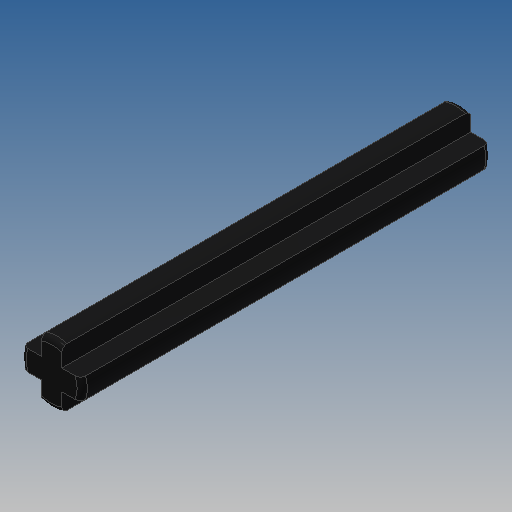
# Autodesk Inventor part: 3705-Black
Saved by Autodesk Inventor 2022.2 (Build 262287000, 287)
## iProperties
Created: 2014-06-05
Part Number: 3705-Black
Material: ABS Plastic
Document SubType Name: Modeling
Designer: D. Kohfeld
Density: 1.06 g/cm^3
Appearance: Black
Mass: 0.423877 g
Surface Area: 6.05529 cm^2
Volume: 0.399884 cm^3
Description: Technic, Axle 4
Author: D. Kohfeld
Autodesk Inventor part; units mm, degrees
ref_plane "YZ Plane" through (0, 0, 0) normal (1, 0, 0) x (0, 1, 0)
ref_plane "XZ Plane" through (0, 0, 0) normal (0, 1, 0) x (-1, 0, 0)
ref_plane "XY Plane" through (0, 0, 0) normal (0, 0, 1) x (1, 0, 0)
sketch "Sketch1" plane through (0, 0, 0) normal (0, 0, 1) x (1, 0, 0)
  circle A0 centre (0, 0) radius 2.4 construction
  line L0 (-0.8, 2.2627) -> (-0.8, 0.8)
  line L1 (-0.8, 0.8) -> (-2.2627, 0.8)
  line L2 (-2.2627, -0.8) -> (-0.8, -0.8)
  line L3 (-0.8, -0.8) -> (-0.8, -2.2627)
  line L4 (0.8, -2.2627) -> (0.8, -0.8)
  line L5 (0.8, -0.8) -> (2.2627, -0.8)
  line L6 (2.2627, 0.8) -> (0.8, 0.8)
  line L7 (0.8, 0.8) -> (0.8, 2.2627)
  arc A1 (0.8, 2.2627) -> (-0.8, 2.2627) centre (0, 0) ccw
  arc A2 (-2.2627, 0.8) -> (-2.2627, -0.8) centre (0, 0) ccw
  arc A3 (-0.8, -2.2627) -> (0.8, -2.2627) centre (0, 0) ccw
  arc A4 (2.2627, -0.8) -> (2.2627, 0.8) centre (0, 0) ccw
  dimension "d0" = 4.8
  dimension "d1" = 1.6
  constraints: 16 end point, 8 point on circle, 7 equal length, 4 centre point, 4 perpendicular, 3 parallel, 1 coincident, 1 vertical, 14 other
  measures "d1" distance between parallel lines of L0 L7
extrude "Extrusion1" add sketch "Sketch1" along normal mid plane 32
fillet "Fillet1" radius 0.4 8 edges at (0, 2.4, 16) (-2.4, 0, 16) (0, -2.4, 16) (2.4, 0, 16) (2.4, 0, -16) (0, 2.4, -16) (-2.4, 0, -16) (0, -2.4, -16)
equation "\"d0\" = kd"
equation "\"d1\" = axlet"
equation "\"d2\" = 4 * lu"
equation "\"d4\" = tf"
equation "\"kd\" = 4.8"
equation "\"axlet\" = 1.6"
equation "\"lu\" = 8"
equation "\"tf\" = 0.4"
body "Solid1"
